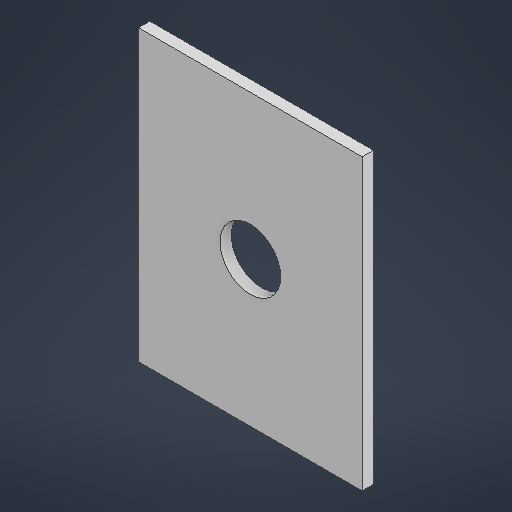
# Autodesk Inventor part: MotorProtector
Saved by Autodesk Inventor 2026.1 (Build 301233000, 233)
## iProperties
Created: 2026-07-02
Part Number: MotorProtector
Material: Generic
Document SubType Name: Modeling
Designer: Kasi Pusuluri
Density: 1 g/cm^3
Appearance: Default
Author: Kasi Pusuluri
Autodesk Inventor part; units mm, degrees
ref_plane "YZ Plane" through (0, 0, 0) normal (1, 0, 0) x (0, 1, 0)
ref_plane "XZ Plane" through (0, 0, 0) normal (0, 1, 0) x (-1, 0, 0)
ref_plane "XY Plane" through (0, 0, 0) normal (0, 0, 1) x (1, 0, 0)
sketch "Sketch1" plane through (0, 0, 0) normal (0, 0, 1) x (1, 0, 0)
  circle A0 centre (0, 0) radius 2
  line L0 (0, 0) -> (7.366, 0)
  line L1 (0, 0) -> (-7.366, 0)
  line L2 (7.366, 0) -> (7.366, 9.525)
  line L3 (-7.366, 0) -> (-7.366, -9.525)
  line L4 (-7.366, -9.525) -> (7.366, -9.525)
  line L5 (7.366, -9.525) -> (7.366, 9.525)
  line L6 (7.366, 9.525) -> (-7.366, 9.525)
  line L7 (-7.366, 9.525) -> (-7.366, -9.525)
  point P0 (7.366, 0)
  dimension "d0" = 4
  dimension "d1" = 7.366
  dimension "d2" = 7.366
  dimension "d3" = 9.525
  dimension "d4" = 9.525
  constraints: 16 end point, 3 horizontal, 2 parallel, 2 vertical, 1 centre point, 1 coincident, 1 perpendicular
  measures "d0" diameter of A0
  measures "d1" distance of L0.start L0.end
  measures "d2" distance of L0.start L1.end
  measures "d3" distance of L0.end L2.end
  measures "d4" distance of L1.end L3.end
extrude "Extrusion1" add sketch "Sketch1" along normal blind 0.75 contours L0 L5 L4 L3 L1 A0 | A0 L1 L7 L6 L2 L0
equation "\"d2\" = d1"
equation "\"d4\" = d3"
body "Solid1"
